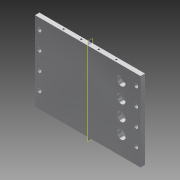
# Autodesk Inventor part: YagiFrontPanel
Saved by Autodesk Inventor 2014 (Build 180170000, 170)
## iProperties
Created: 2015-05-19
Part Number: YagiFrontPanel
Material: Generic
Document SubType Name: Modeling
Designer: Owner
Density: 1 g/cm^3
Appearance: Aluminum - Polished
Author: Owner
Autodesk Inventor part; units mm, degrees
ref_plane "YZ Plane" through (0, 0, 0) normal (1, 0, 0) x (0, 1, 0)
ref_plane "XZ Plane" through (0, 0, 0) normal (0, 1, 0) x (-1, 0, 0)
ref_plane "XY Plane" through (0, 0, 0) normal (0, 0, 1) x (1, 0, 0)
sketch "Sketch1" plane through (0, 0, 0) normal (0, 0, 1) x (1, 0, 0)
  line L0 (-72.6181, 62.4032) -> (3.5819, 62.4032)
  line L1 (3.5819, 62.4032) -> (3.5819, 5.2532)
  line L2 (3.5819, 5.2532) -> (-72.6181, 5.2532)
  line L3 (-72.6181, 5.2532) -> (-72.6181, 62.4032)
  point P0 (0, 0)
  dimension "d0" = 76.2
  dimension "d1" = 57.15
  constraints: 8 end point, 2 parallel, 1 horizontal, 1 perpendicular
  measures "d0" distance of L0.start L0.end
  measures "d1" distance of L0.end L1.end
extrude "Extrusion1" add sketch "Sketch1" along normal blind 3.175
sketch "Sketch5" plane through (0, 0, 3.175) normal (0, 0, 1) x (1, 0, 0)
  line L0 (3.5819, 62.4032) -> (-72.6181, 62.4032) projected
  circle A0 centre (-10.3881, 52.2432) radius 3.175
  line L1 (3.5819, 5.2532) -> (3.5819, 62.4032) projected
  circle A1 centre (-10.3881, 40.8132) radius 3.175
  circle A2 centre (-10.3881, 29.3832) radius 3.175
  circle A3 centre (-10.3881, 17.9532) radius 3.175
  point P0 (0, 0)
  dimension "d48" = 6.35
  dimension "d49" = 13.97
  dimension "d50" = 10.16
  dimension "d53" = 11.43
  constraints: 4 centre point, 1 vertical, 6 other
  measures "d48" diameter of A0
  measures "d49" distance from line of L1 A0.centre
  measures "d50" distance from line of L0 A0.centre
  measures "d53" distance of A0.centre A1.centre
sketch "Sketch2" plane through (-72.6181, 62.4032, 0) normal (0, 1, 0) x (1, 0, 0)
  point P0 (57.15, -1.5875)
hole "Hole1" at (-15.4681, 62.4032, 1.5875) direction (0, -1, 0) diameter 1.1811 depth 4.699 tip angle 120 thread size "0-80 UNF" class "2B" standard "ANSI Unified Screw Threads"
sketch "Sketch3" plane through (-72.6181, 5.2532, 0) normal (0, -1, 0) x (1, 0, 0)
  point P0 (19.05, 1.5875)
hole "Hole3" at (-53.5681, 5.2532, 1.5875) direction (0, 1, 0) diameter 1.1811 depth 4.699 tip angle 120 thread size "0-80 UNF" class "2B" standard "ANSI Unified Screw Threads"
pattern_linear "Rectangular Pattern1" count 2 spacing 12.7 along (1, 0, 0) of "Hole3"
pattern_linear "Rectangular Pattern2" count 2 spacing 12.7 along (-1, 0, 0) of "Hole1"
ref_plane "Work Plane1" through (-34.5181, 5.2532, 0) normal (-1, 0, 0) x (0, 0, 1)
sketch "Sketch4" plane through (0, 0, 3.175) normal (0, 0, 1) x (1, 0, 0)
  point P0 (0.4069, 54.7832)
hole "Hole5" at (0.4069, 54.7832, 3.175) direction (0, 0, -1) diameter 1.778 depth 3.175 countersink diameter 3.0226 countersink angle 82
pattern_linear "Rectangular Pattern3" count 4 spacing 12.7 along (0, -1, 0) of "Hole5"
extrude "Extrusion3" cut sketch "Sketch5" against normal up to next
mirror "Mirror1" about plane through (-34.5181, 5.2532, 0) normal (-1, 0, 0) of "Hole3", "Rectangular Pattern1", "Hole5", "Rectangular Pattern3", "Hole1", "Rectangular Pattern2", "Extrusion3"
body "Solid1"
